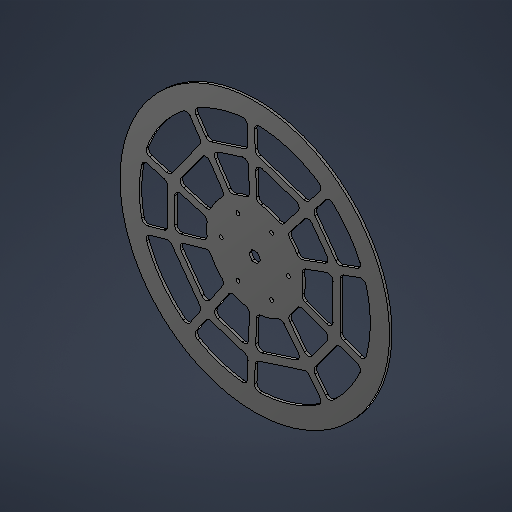
# Autodesk Inventor part: PLATE,BOTTOM
Saved by Autodesk Inventor 2026 (Build 300175000, 175)
## iProperties
Created: 2026-02-06
Part Number: PLATE,BOTTOM
Material: Nylon, molybdenum disulphide
Document SubType Name: Sheet Metal
Designer: littl
Density: 1.13 g/cm^3
Sheet Metal Rule: Default
Appearance: Smooth - Black
Mass: 193.014 g
Surface Area: 1234 cm^2
Volume: 170.809 cm^3
Author: littl
Autodesk Inventor part; units mm, degrees
ref_plane "YZ Plane" through (0, 0, 0) normal (1, 0, 0) x (0, 1, 0)
ref_plane "XZ Plane" through (0, 0, 0) normal (0, 1, 0) x (-1, 0, 0)
ref_plane "XY Plane" through (0, 0, 0) normal (0, 0, 1) x (1, 0, 0)
sketch "Sketch1" plane through (0, 0, 0) normal (0, 0, 1) x (1, 0, 0)
  circle A0 centre (0, 0) radius 177.8
  dimension "d0" = 355.6
  measures "d0" diameter of A0
extrude "Plate1" add sketch "Sketch1" along normal blind 3.175
sketch "Sketch2" plane through (0, 0, 3.175) normal (0, 0, 1) x (1, 0, 0)
  line L0 (3.7395, -6.477) -> (-3.7395, -6.477)
  line L1 (-3.7395, -6.477) -> (-7.479, 0)
  line L2 (-7.479, 0) -> (-3.7395, 6.477)
  line L3 (-3.7395, 6.477) -> (3.7395, 6.477)
  line L4 (3.7395, 6.477) -> (7.479, 0)
  line L5 (7.479, 0) -> (3.7395, -6.477)
  point P0 (0, 0)
  point P1 (0, 0)
  dimension "d2" = 12.954
  constraints: 12 end point, 1 coincident, 1 horizontal, 13 other
  measures "d2" distance between parallel lines of L3 L0
extrude "Cut1" cut sketch "Sketch2" against normal blind 3.175
sketch "Sketch3" plane through (0, 0, 3.175) normal (0, 0, 1) x (1, 0, 0)
  point P0 (0, 0)
  point P1 (-44.45, 0)
  point P2 (-22.225, -38.4948)
  point P3 (22.225, -38.4948)
  point P4 (44.45, 0)
  point P5 (22.225, 38.4948)
  point P6 (-22.225, 38.4948)
  dimension "d5" = 44.45
  dimension "d8" = 360
  constraints: 1 horizontal alignment, 7 other
  measures "d5" distance of point (-44.45, 0) point (0, 0)
hole "Hole1" at (-44.45, 0, 3.175) at (-22.225, -38.4948, 3.175) at (22.225, -38.4948, 3.175) at (44.45, 0, 3.175) at (22.225, 38.4948, 3.175) at (-22.225, 38.4948, 3.175) direction (0, 0, -1) diameter 5.1054 end through all clearance for "Flat Head Machine Screw (82)" size "#10" standard "Ansi Unified Screw Threads"
sketch "Sketch4" plane through (0, 0, 3.175) normal (0, 0, 1) x (1, 0, 0)
  circle A0 centre (0, 0) radius 152.4
  circle A1 centre (0, 0) radius 63.5
  line L0 (0, 0) -> (167.0773, 60.8112) construction
  circle A2 centre (0, 0) radius 177.8 projected
  line L1 (-1.6289, 4.4753) -> (165.4485, 65.2865)
  line L2 (168.7062, 56.3359) -> (1.6289, -4.4753)
  arc A3 (-1.6289, 4.4753) -> (1.6289, -4.4753) centre (0, 0) ccw
  arc A4 (168.7062, 56.3359) -> (165.4485, 65.2865) centre (167.0773, 60.8112) ccw
  line L3 (0, 0) -> (167.0773, -60.8112) construction
  line L4 (-1.6289, -4.4753) -> (165.4485, -65.2865)
  line L5 (168.7062, -56.3359) -> (1.6289, 4.4753)
  arc A5 (1.6289, 4.4753) -> (-1.6289, -4.4753) centre (0, 0) ccw
  arc A6 (165.4485, -65.2865) -> (168.7062, -56.3359) centre (167.0773, -60.8112) ccw
  line L6 (107.95, 39.2906) -> (107.95, -39.2906) construction
  line L7 (103.1875, 39.2906) -> (103.1875, -39.2906)
  line L8 (112.7125, -39.2906) -> (112.7125, 39.2906)
  arc A7 (112.7125, 39.2906) -> (103.1875, 39.2906) centre (107.95, 39.2906) ccw
  arc A8 (103.1875, -39.2906) -> (112.7125, -39.2906) centre (107.95, -39.2906) ccw
  line L9 (-5.4809, 110.2786) -> (69.2543, 85.9957)
  line L10 (-4.0092, 114.808) -> (70.726, 90.5251) construction
  line L11 (72.1976, 95.0545) -> (-2.5375, 119.3374)
  arc A9 (-2.5375, 119.3374) -> (-5.4809, 110.2786) centre (-4.0092, 114.808) ccw
  arc A10 (69.2543, 85.9957) -> (72.1976, 95.0545) centre (70.726, 90.5251) ccw
  line L12 (-1.4455, 177.8579) -> (4.7596, 0.1662)
  line L13 (0, 0) -> (-6.2051, 177.6917) construction
  line L14 (-4.7596, -0.1662) -> (-10.9647, 177.5255)
  line L15 (105.7117, 143.0404) -> (-3.7529, 2.9321)
  line L16 (0, 0) -> (109.4646, 140.1083) construction
  line L17 (3.7529, -2.9321) -> (113.2175, 137.1762)
  line L18 (-106.5749, 28.8653) -> (-60.386, 92.4388)
  line L19 (-110.4278, 31.6647) -> (-64.239, 95.2382) construction
  line L20 (-68.0919, 98.0375) -> (-114.2808, 34.464)
  arc A11 (-114.2808, 34.464) -> (-106.5749, 28.8653) centre (-110.4278, 31.6647) ccw
  arc A12 (-60.386, 92.4388) -> (-68.0919, 98.0375) centre (-64.239, 95.2382) ccw
  line L21 (-169.5996, 53.5863) -> (1.3127, 4.578)
  line L22 (0, 0) -> (-170.9123, 49.0083) construction
  line L23 (-1.3127, -4.578) -> (-172.2251, 44.4303)
  line L24 (-103.3728, 144.7397) -> (-3.9483, -2.6632)
  line L25 (0, 0) -> (-99.4245, 147.4029) construction
  line L26 (3.9483, 2.6632) -> (-95.4762, 150.066)
  line L27 (-60.386, -92.4388) -> (-106.5749, -28.8653)
  line L28 (-64.239, -95.2382) -> (-110.4278, -31.6647) construction
  line L29 (-114.2808, -34.464) -> (-68.0919, -98.0375)
  arc A13 (-68.0919, -98.0375) -> (-60.386, -92.4388) centre (-64.239, -95.2382) ccw
  arc A14 (-106.5749, -28.8653) -> (-114.2808, -34.464) centre (-110.4278, -31.6647) ccw
  line L30 (-103.3728, -144.7397) -> (-3.9483, 2.6632)
  line L31 (0, 0) -> (-99.4245, -147.4029) construction
  line L32 (3.9483, -2.6632) -> (-95.4762, -150.066)
  line L33 (-169.5996, -53.5863) -> (1.3127, -4.578)
  line L34 (0, 0) -> (-170.9123, -49.0083) construction
  line L35 (-1.3127, 4.578) -> (-172.2251, -44.4303)
  line L36 (69.2543, -85.9957) -> (-5.4809, -110.2786)
  line L37 (70.726, -90.5251) -> (-4.0092, -114.808) construction
  line L38 (-2.5375, -119.3374) -> (72.1976, -95.0545)
  arc A15 (72.1976, -95.0545) -> (69.2543, -85.9957) centre (70.726, -90.5251) ccw
  arc A16 (-5.4809, -110.2786) -> (-2.5375, -119.3374) centre (-4.0092, -114.808) ccw
  line L39 (105.7117, -143.0404) -> (-3.7529, -2.9321)
  line L40 (0, 0) -> (109.4646, -140.1083) construction
  line L41 (3.7529, 2.9321) -> (113.2175, -137.1762)
  line L42 (-1.4455, -177.8579) -> (4.7596, -0.1662)
  line L43 (0, 0) -> (-6.2051, -177.6917) construction
  line L44 (-4.7596, 0.1662) -> (-10.9647, -177.5255)
  line L45 (107.95, 39.2906) -> (70.726, 90.5251) construction
  line L46 (111.8029, 42.0899) -> (74.5789, 93.3244)
  line L47 (66.873, 87.7258) -> (104.0971, 36.4913)
  arc A17 (104.0971, 36.4913) -> (111.8029, 42.0899) centre (107.95, 39.2906) ccw
  arc A18 (74.5789, 93.3244) -> (66.873, 87.7258) centre (70.726, 90.5251) ccw
  line L48 (-4.0092, 114.808) -> (-64.239, 95.2382) construction
  line L49 (-2.5375, 110.2786) -> (-62.7673, 90.7088)
  line L50 (-65.7107, 99.7676) -> (-5.4809, 119.3374)
  arc A19 (-2.5375, 110.2786) -> (-5.4809, 119.3374) centre (-4.0092, 114.808) ccw
  arc A20 (-65.7107, 99.7676) -> (-62.7673, 90.7088) centre (-64.239, 95.2382) ccw
  line L51 (70.726, -90.5251) -> (107.95, -39.2906) construction
  line L52 (66.873, -87.7258) -> (104.0971, -36.4913)
  line L53 (111.8029, -42.0899) -> (74.5789, -93.3244)
  arc A21 (66.873, -87.7258) -> (74.5789, -93.3244) centre (70.726, -90.5251) ccw
  arc A22 (111.8029, -42.0899) -> (104.0971, -36.4913) centre (107.95, -39.2906) ccw
  line L54 (-4.0092, -114.808) -> (-64.239, -95.2382) construction
  line L55 (-2.5375, -110.2786) -> (-62.7673, -90.7088)
  line L56 (-65.7107, -99.7676) -> (-5.4809, -119.3374)
  arc A23 (-5.4809, -119.3374) -> (-2.5375, -110.2786) centre (-4.0092, -114.808) ccw
  arc A24 (-62.7673, -90.7088) -> (-65.7107, -99.7676) centre (-64.239, -95.2382) ccw
  line L57 (-110.4278, -31.6647) -> (-110.4278, 31.6647) construction
  line L58 (-115.1903, -31.6647) -> (-115.1903, 31.6647)
  line L59 (-105.6653, 31.6647) -> (-105.6653, -31.6647)
  arc A25 (-115.1903, -31.6647) -> (-105.6653, -31.6647) centre (-110.4278, -31.6647) ccw
  arc A26 (-105.6653, 31.6647) -> (-115.1903, 31.6647) centre (-110.4278, 31.6647) ccw
  point P0 (83.5387, 30.4056)
  point P1 (83.5387, -30.4056)
  point P2 (107.95, 0)
  point P3 (33.3584, 102.6666)
  point P4 (-3.1026, 88.8458)
  point P5 (54.7323, 70.0542)
  point P6 (-87.3334, 63.4514)
  point P7 (-85.4562, 24.5042)
  point P8 (-49.7122, 73.7014)
  point P9 (-87.3334, -63.4514)
  point P10 (-49.7122, -73.7014)
  point P11 (-85.4562, -24.5042)
  point P12 (33.3584, -102.6666)
  point P13 (54.7323, -70.0542)
  point P14 (-3.1026, -88.8458)
  point P15 (89.338, 64.9078)
  point P16 (-34.1241, 105.0231)
  point P17 (89.338, -64.9078)
  point P18 (-34.1241, -105.0231)
  point P19 (-110.4278, 0)
  point P20 (100.3822, 41.6043)
  point P21 (70.5878, 82.6127)
  point P22 (42.7373, 46.9657)
  point P23 (57.8736, 26.1324)
  point P24 (76.6883, 90.421)
  point P25 (109.6935, 44.9933)
  point P26 (141.5103, 56.5737)
  point P27 (97.5339, 117.1021)
  point P28 (35.2315, 52.8298)
  point P29 (62.7856, 88.0975)
  point P30 (0.9878, 108.1768)
  point P31 (2.5497, 63.4488)
  point P32 (69.0261, 96.085)
  point P33 (90.0281, 122.9663)
  point P34 (-0.5565, 152.399)
  point P35 (0.634, 118.3069)
  point P36 (-8.5482, 108.3256)
  point P37 (-56.7565, 92.6618)
  point P38 (-31.4604, 55.1588)
  point P39 (-6.9695, 63.1164)
  point P40 (-62.2975, 100.8766)
  point P41 (-8.894, 118.2284)
  point P42 (-10.0757, 152.0666)
  point P43 (-81.2311, 128.9468)
  point P44 (-39.357, 49.8325)
  point P45 (-64.3839, 86.9363)
  point P46 (-102.577, 34.3679)
  point P47 (-59.5555, 22.0317)
  point P48 (-70.052, 95.3396)
  point P49 (-89.1277, 123.6205)
  point P50 (-145.112, 46.5646)
  point P51 (-112.3206, 37.1619)
  point P52 (-115.1903, -28.0759)
  point P53 (-115.1903, 28.0759)
  point P54 (-147.7375, 37.4086)
  point P55 (-147.7375, -37.4086)
  point P56 (-105.6653, 25.3446)
  point P57 (-105.6653, -25.3446)
  point P58 (-62.1809, -12.8757)
  point P59 (-62.1809, 12.8757)
  point P60 (-112.3206, -37.1619)
  point P61 (-145.112, -46.5646)
  point P62 (-89.1277, -123.6205)
  point P63 (-70.052, -95.3396)
  point P64 (-59.5555, -22.0317)
  point P65 (-102.577, -34.3679)
  point P66 (-64.3839, -86.9363)
  point P67 (-39.357, -49.8325)
  point P68 (-8.894, -118.2284)
  point P69 (-62.2975, -100.8766)
  point P70 (-81.2311, -128.9468)
  point P71 (-10.0757, -152.0666)
  point P72 (-56.7565, -92.6618)
  point P73 (-8.5482, -108.3256)
  point P74 (-6.9695, -63.1164)
  point P75 (-31.4604, -55.1588)
  point P76 (2.5497, -63.4488)
  point P77 (0.9878, -108.1768)
  point P78 (62.7856, -88.0975)
  point P79 (35.2315, -52.8298)
  point P80 (0.634, -118.3069)
  point P81 (-0.5565, -152.399)
  point P82 (90.0281, -122.9663)
  point P83 (69.0261, -96.085)
  point P84 (100.3822, -41.6043)
  point P85 (109.6935, -44.9933)
  point P86 (76.6883, -90.421)
  point P87 (97.5339, -117.1021)
  point P88 (141.5103, -56.5737)
  point P89 (70.5878, -82.6127)
  point P90 (57.8736, -26.1324)
  point P91 (42.7373, -46.9657)
  point P92 (103.1875, -32.489)
  point P93 (103.1875, 32.489)
  point P94 (61.1313, 17.1818)
  point P95 (61.1313, -17.1818)
  point P96 (112.7125, 35.9558)
  point P97 (112.7125, -35.9558)
  point P98 (144.7681, -47.6231)
  point P99 (144.7681, 47.6231)
  dimension "d17" = 304.8
  dimension "d18" = 127
  dimension "d19" = 40
  dimension "d20" = 107.95
  dimension "d21" = 4.7625
  dimension "d24" = 360
  constraints: 160 end point, 50 point on circle, 32 tangent, 26 centre point, 10 point on line, 8 midpoint, 8 parallel, 7 equal radius, 2 coincident, 2 vertical, 1 horizontal alignment, 156 other
  measures "d17" diameter of A0
  measures "d18" diameter of A1
  measures "d19" angle of L3 L0
  measures "d20" distance of point (0, 0) point (107.95, 0)
  measures "d21" radius of A8
extrude "Cut2" cut sketch "Sketch4" against normal blind 3.175 contours A0 L5 L8 L2 | L1 L46 L17 A0 | A0 L41 L53 L4 | L15 L11 L12 A0 | L7 L5 A1 L2 | A0 L42 L38 L39 | L1 A1 L17 L47 | L52 L41 A1 L4 | L14 L50 L26 A0 | A0 L32 L56 L44 | L15 A1 L12 L9 | L36 L42 A1 L39 | L24 L20 L21 A0 | A0 L33 L29 L30 | L14 A1 L26 L49 | L55 L32 A1 L44 | L23 L58 L35 A0 | L24 A1 L21 L18 | L27 L33 A1 L30 | L23 A1 L35 L59
fillet "Corner Round1" radius 6.35 80 edges at (-62.1809, -12.8757, 1.5875) (0.634, -118.3069, 1.5875) (-0.5565, -152.399, 1.5875) (90.0281, -122.9663, 1.5875) (69.0261, -96.085, 1.5875) (-39.357, 49.8325, 1.5875) (-64.3839, 86.9363, 1.5875) (-115.1903, 28.0759, 1.5875) (-112.3206, 37.1619, 1.5875) (-145.112, 46.5646, 1.5875) (-70.052, 95.3396, 1.5875) (-89.1277, 123.6205, 1.5875) (-56.7565, 92.6618, 1.5875) (-31.4604, 55.1588, 1.5875) (-6.9695, 63.1164, 1.5875) (57.8736, 26.1324, 1.5875) (-8.5482, 108.3256, 1.5875) (-62.2975, 100.8766, 1.5875) (-81.2311, 128.9468, 1.5875) (-39.357, -49.8325, 1.5875) (-59.5555, -22.0317, 1.5875) (-64.3839, -86.9363, 1.5875) (-102.577, -34.3679, 1.5875) (-115.1903, -28.0759, 1.5875) (100.3822, -41.6043, 1.5875) (70.5878, -82.6127, 1.5875) (42.7373, -46.9657, 1.5875) (61.1313, -17.1818, 1.5875) (61.1313, 17.1818, 1.5875) (76.6883, -90.421, 1.5875) (97.5339, -117.1021, 1.5875) (103.1875, -32.489, 1.5875) (109.6935, -44.9933, 1.5875) (141.5103, -56.5737, 1.5875) (103.1875, 32.489, 1.5875) (57.8736, -26.1324, 1.5875) (112.7125, 35.9558, 1.5875) (112.7125, -35.9558, 1.5875) (144.7681, -47.6231, 1.5875) (144.7681, 47.6231, 1.5875) (62.7856, 88.0975, 1.5875) (35.2315, 52.8298, 1.5875) (0.9878, 108.1768, 1.5875) (2.5497, 63.4488, 1.5875) (76.6883, 90.421, 1.5875) (-8.894, 118.2284, 1.5875) (-10.0757, 152.0666, 1.5875) (90.0281, 122.9663, 1.5875) (42.7373, 46.9657, 1.5875) (100.3822, 41.6043, 1.5875) (70.5878, 82.6127, 1.5875) (69.0261, 96.085, 1.5875) (-0.5565, 152.399, 1.5875) (0.634, 118.3069, 1.5875) (97.5339, 117.1021, 1.5875) (109.6935, 44.9933, 1.5875) (141.5103, 56.5737, 1.5875) (-147.7375, 37.4086, 1.5875) (-31.4604, -55.1588, 1.5875) (-6.9695, -63.1164, 1.5875) (-8.5482, -108.3256, 1.5875) (-147.7375, -37.4086, 1.5875) (-62.2975, -100.8766, 1.5875) (-8.894, -118.2284, 1.5875) (-10.0757, -152.0666, 1.5875) (-81.2311, -128.9468, 1.5875) (-56.7565, -92.6618, 1.5875) (-102.577, 34.3679, 1.5875) (-59.5555, 22.0317, 1.5875) (-70.052, -95.3396, 1.5875) (-89.1277, -123.6205, 1.5875) (-112.3206, -37.1619, 1.5875) (-145.112, -46.5646, 1.5875) (-105.6653, -25.3446, 1.5875) (-105.6653, 25.3446, 1.5875) (-62.1809, 12.8757, 1.5875) (62.7856, -88.0975, 1.5875) (35.2315, -52.8298, 1.5875) (2.5497, -63.4488, 1.5875) (0.9878, -108.1768, 1.5875)
equation "\"d3\" = Thickness"
equation "\"d15\" = Thickness"
equation "\"d26\" = Thickness"
equation "\"d1\" = Thickness"
equation "\"BendRadius\" = Thickness"
equation "\"BendReliefWidth\" = Thickness"
equation "\"BendReliefDepth\" = 0.5 * Thickness"
equation "\"CornerReliefSize\" = 4 * Thickness"
equation "\"MinimumRemnant\" = 2 * Thickness"
equation "\"TransitionRadius\" = BendRadius"
equation "\"JacobiRadiusSize\" = BendRadius"
equation "\"GapSize\" = Thickness"
equation "\"Thickness\" = 3.175"
body "Solid1"
